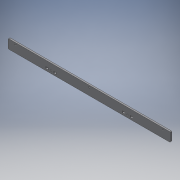
# Autodesk Inventor part: wiper
Saved by Autodesk Inventor 2019 (Build 230136000, 136)
## iProperties
Created: 2020-07-09
Part Number: wiper
Material: Generic
Document SubType Name: Modeling
Designer: Vijay
Density: 1 g/cm^3
Appearance: Default
Author: Vijay
Autodesk Inventor part; units mm, degrees
ref_plane "YZ Plane" through (0, 0, 0) normal (1, 0, 0) x (0, 1, 0)
ref_plane "XZ Plane" through (0, 0, 0) normal (0, 1, 0) x (-1, 0, 0)
ref_plane "XY Plane" through (0, 0, 0) normal (0, 0, 1) x (1, 0, 0)
sketch "Sketch1" plane through (0, 0, 0) normal (0, 0, 1) x (1, 0, 0)
  line L0 (430, 0) -> (430, -4) projected
  line L1 (100, -4) -> (100, 0) construction
  line L2 (0, 0) -> (100, 0) construction
  line L3 (0, 0) -> (0, -4) projected
  line L4 (100, -4) -> (0, -4) construction
  line L5 (0, -9) -> (430, -9)
  line L6 (430, -9) -> (430, 15)
  line L7 (430, 15) -> (0, 15)
  line L8 (0, 15) -> (0, -9)
  line L9 (324, 0) -> (324, -4) construction
  line L10 (330, 0) -> (330, -4) construction
  line L11 (302.8, 0) -> (302.8, -4) construction
  line L12 (308.8, 0) -> (308.8, -4) construction
  line L13 (318.1, -4) -> (314.7, -4) construction
  line L14 (318.1, 0) -> (318.1, -4) construction
  line L15 (314.7, 0) -> (318.1, 0) construction
  line L16 (314.7, 0) -> (314.7, -4) construction
  line L17 (106, 0) -> (106, -4) construction
  line L18 (100, 0) -> (100, -4) construction
  line L19 (121.2, 0) -> (121.2, -4) construction
  line L20 (127.2, 0) -> (127.2, -4) construction
  line L21 (100, 0) -> (106, 0) construction
  line L22 (106, 0) -> (106, -4) construction
  line L23 (106, -4) -> (100, -4) construction
  line L24 (100, -4) -> (100, 0) construction
  line L25 (121.2, 0) -> (127.2, 0) construction
  line L26 (127.2, 0) -> (127.2, -4) construction
  line L27 (127.2, -4) -> (121.2, -4) construction
  line L28 (121.2, -4) -> (121.2, 0) construction
  line L29 (302.8, 0) -> (308.8, 0) construction
  line L30 (308.8, 0) -> (308.8, -4) construction
  line L31 (308.8, -4) -> (302.8, -4) construction
  line L32 (302.8, -4) -> (302.8, 0) construction
  line L33 (324, 0) -> (330, 0) construction
  line L34 (330, 0) -> (330, -4) construction
  line L35 (330, -4) -> (324, -4) construction
  line L36 (324, -4) -> (324, 0) construction
  line L37 (115.3, -4) -> (111.9, -4) construction
  line L38 (115.3, 0) -> (115.3, -4) construction
  line L39 (111.9, 0) -> (115.3, 0) construction
  line L40 (111.9, 0) -> (111.9, -4) construction
  line L41 (106.2, 0.2) -> (99.8, 0.2)
  line L42 (99.8, 0.2) -> (99.8, -4.2)
  line L43 (99.8, -4.2) -> (106.2, -4.2)
  line L44 (106.2, -4.2) -> (106.2, 0.2)
  line L45 (127.4, 0.2) -> (121, 0.2)
  line L46 (121, 0.2) -> (121, -4.2)
  line L47 (121, -4.2) -> (127.4, -4.2)
  line L48 (127.4, -4.2) -> (127.4, 0.2)
  line L49 (309, 0.2) -> (302.6, 0.2)
  line L50 (302.6, 0.2) -> (302.6, -4.2)
  line L51 (302.6, -4.2) -> (309, -4.2)
  line L52 (309, -4.2) -> (309, 0.2)
  line L53 (330.2, 0.2) -> (323.8, 0.2)
  line L54 (323.8, 0.2) -> (323.8, -4.2)
  line L55 (323.8, -4.2) -> (330.2, -4.2)
  line L56 (330.2, -4.2) -> (330.2, 0.2)
  circle A0 centre (316.4, -2) radius 1.6
  circle A1 centre (113.6, -2) radius 1.6
  dimension "d0" = 5
  dimension "d1" = 15
  dimension "d2" = 0.2
  dimension "d3" = 0.2
  dimension "d4" = 0.2
  dimension "d5" = 0.2
  dimension "d6" = 3.2
  dimension "d7" = 3.2
  constraints: 72 end point, 18 parallel, 9 perpendicular, 5 horizontal, 2 centre point, 12 other
  measures "d0" distance between parallel lines of L5 L4
  measures "d1" distance between parallel lines of L2 L7
  measures "d2" distance between parallel lines of L21 L41
  measures "d3" distance between parallel lines of L25 L45
  measures "d4" distance between parallel lines of L29 L49
  measures "d5" distance between parallel lines of L33 L53
  measures "d6" diameter of A0
  measures "d7" diameter of A1
extrude "Extrusion1" add sketch "Sketch1" along normal blind 4
fillet "Fillet1" radius 2 4 edges at (0, 15, 2) (0, -9, 2) (430, 15, 2) (430, -9, 2)
sketch "Sketch2" plane through (0, 0, 4) normal (0, 0, 1) x (1, 0, 0)
  circle A0 centre (20, 7) radius 2
  circle A1 centre (215, 7) radius 2
  circle A2 centre (410, 7) radius 2
  line L0 (0, 13) -> (0, -7) projected
  line L1 (430, -7) -> (430, 13) projected
  line L2 (428, 15) -> (2, 15) projected
  point P0 (0, 0)
  dimension "d11" = 4
  dimension "d12" = 4
  dimension "d13" = 4
  dimension "d14" = 20
  dimension "d15" = 20
  dimension "d16" = 8
  dimension "d17" = 8
  dimension "d18" = 8
  constraints: 3 centre point
  measures "d11" diameter of A0
  measures "d12" diameter of A1
  measures "d13" diameter of A2
  measures "d14" distance from line of L0 A0.centre
  measures "d15" distance from line of L1 A2.centre
  measures "d16" distance from line of A0.centre L2
  measures "d17" distance from line of A1.centre L2
  measures "d18" distance from line of A2.centre L2
extrude "Extrusion2" cut sketch "Sketch2" against normal blind 4
body "Solid1"
